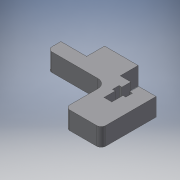
# Autodesk Inventor part: A8-0017
Saved by Autodesk Inventor 2016 SP2 (Build 200236200, 236)
## iProperties
Created: 2017-04-22
Part Number: A8-0017
Material: Generic
Document SubType Name: Modeling
Designer: EV
Density: 1 g/cm^3
Appearance: Default
Author: EV
Autodesk Inventor part; units mm, degrees
ref_plane "YZ Plane" through (0, 0, 0) normal (1, 0, 0) x (0, 1, 0)
sketch "Sketch1" plane through (0, 0, 0) normal (0, 1, 0) x (-1, 0, 0)
  line L0 (0, 0) -> (16, 0)
  line L1 (16, 0) -> (16, -18.5)
  line L2 (0, -24.5) -> (0, 0)
  line L3 (0, -24.5) -> (16, -24.5)
  line L4 (11.25, -24.5) -> (11.25, -20.5)
  line L5 (11.25, -20.5) -> (12.5, -20.5)
  line L6 (12.5, -20.5) -> (12.5, -17.5)
  line L7 (12.5, -17.5) -> (11.25, -17.5)
  line L8 (11.25, -17.5) -> (11.25, -12.5)
  line L9 (11.25, -12.5) -> (7.75, -12.5)
  line L10 (7.75, -12.5) -> (7.75, -17.5)
  line L11 (7.75, -17.5) -> (6.5, -17.5)
  line L12 (6.5, -17.5) -> (6.5, -20.5)
  line L13 (6.5, -20.5) -> (7.75, -20.5)
  line L14 (7.75, -24.5) -> (7.75, -20.5)
  line L15 (16, -18.5) -> (42.5, -18.5)
  line L16 (42.5, -18.5) -> (42.5, -24.5)
  line L17 (42.5, -24.5) -> (31, -24.5)
  line L18 (31, -24.5) -> (31, -32.5)
  line L19 (31, -32.5) -> (16, -32.5)
  line L20 (16, -32.5) -> (16, -24.5)
  line L21 (9.5, -12.5) -> (9.5, -24.5) construction
  dimension "d0" = 24.5
  dimension "d1" = 16
  dimension "d4" = 3.5
  dimension "d5" = 6
  dimension "d6" = 4
  dimension "d7" = 3
  dimension "d8" = 5
  dimension "d23" = 7.75
  dimension "d24" = 6
  dimension "d25" = 14
  dimension "d26" = 42.5
  dimension "d27" = 11.5
  dimension "d28" = 15
  dimension "d29" = 32.5
  constraints: 44 end point, 17 perpendicular, 10 point on line, 2 horizontal, 1 collinear, 1 midpoint, 1 parallel
  measures "d0" distance of L2.start L0.start
  measures "d1" distance between parallel lines of L2 L1
  measures "d4" distance between parallel lines of L14 L4
  measures "d5" distance between parallel lines of L12 L6
  measures "d6" distance of L14.start L13.end
  measures "d7" distance of L11.end L12.end
  measures "d8" distance of L9.end L10.end
  measures "d23" distance between parallel lines of L2 L14
  measures "d24" distance between parallel lines of L17 L15
  measures "d25" distance between parallel lines of L19 L15
  measures "d26" distance between parallel lines of L2 L16
  measures "d27" distance between parallel lines of L16 L18
  measures "d28" distance of L18.end L19.end
  measures "d29" distance between parallel lines of L0 L19
extrude "Extrusion1" add sketch "Sketch1" along normal blind 8 contours L0 L1 L15 L16 L17 L18 L19 L20 L3 L4 L5 L6 L7 L8 L9 L10 L11 L12 L13 L14 L2
fillet "Fillet1" radius 2 3 edges at (-16, 4, 0) (0, 4, 0) (-42.5, 4, -18.5)
fillet "Fillet2" radius 4 1 edges at (-16, 4, -18.5)
ref_plane "Work Plane1" through (0, 4, 0) normal (0, 1, 0) x (-1, 0, 0)
ref_plane "Work Plane2" through (-9.5, 0, -12.5) normal (1, 0, 0) x (0, 0, -1)
equation "\"d31\" = 0.5 * THICKNESS"
equation "\"THICKNESS\" = 8"
body "Solid1"
